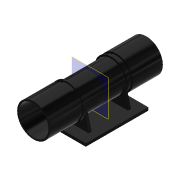
# Autodesk Inventor part: 00_Sensirion_Flowsensor
Saved by Autodesk Inventor 2019.4 (Build 234330000, 330)
## iProperties
Created: 2021-06-01
Part Number: 00_Sensirion_Flowsensor
Material: Generic
Document SubType Name: Modeling
Designer: diederichbenedict
Density: 1 g/cm^3
Appearance: Smooth - Black
Author: diederichbenedict
Autodesk Inventor part; units mm, degrees
ref_plane "YZ Plane" through (0, 0, 0) normal (1, 0, 0) x (0, 1, 0)
ref_plane "XZ Plane" through (0, 0, 0) normal (0, 1, 0) x (-1, 0, 0)
ref_plane "XY Plane" through (0, 0, 0) normal (0, 0, 1) x (1, 0, 0)
sketch "Sketch1" plane through (0, 0, 0) normal (0, 1, 0) x (-1, 0, 0)
  line L0 (0, 0) -> (0, 17.6)
  line L1 (0, 17.6) -> (0, 37.6)
  line L2 (0, 37.6) -> (11, 37.6)
  line L3 (11, 37.6) -> (11, 17.6)
  line L4 (11, 17.6) -> (9.9, 17.6)
  line L5 (9.9, 17.6) -> (9.9, 15.1)
  line L6 (9.9, 15.1) -> (11, 15.1)
  line L7 (11, 15.1) -> (11, 14.1)
  line L8 (11, 14.1) -> (9.9, 14.1)
  line L9 (9.9, 14.1) -> (9.9, 0)
  line L10 (9.9, 0) -> (0, 0)
  dimension "d0" = 17.6
  dimension "d1" = 20
  dimension "d2" = 11
  dimension "d3" = 20
  dimension "d4" = 9.9
  dimension "d6" = 2.5
  dimension "d7" = 1
  dimension "d8" = 0
  constraints: 22 end point, 6 perpendicular, 2 point on line, 1 parallel, 1 vertical
  measures "d0" distance of L0.start L0.end
  measures "d1" distance of L0.end L1.end
  measures "d2" distance of L1.end L2.end
  measures "d3" distance of L2.end L3.end
  measures "d4" distance of L9.end L0.start
  measures "d6" distance between parallel lines of L6 L4
  measures "d7" distance between parallel lines of L8 L6
  measures "d8" distance between parallel lines of L7 L3
revolve "Revolution1" add sketch "Sketch1" angle 360 about axis through (0, 0, 17.6) along (0, 0, 1)
sketch "Sketch2" plane through (0, 0, 37.6) normal (0, 0, 1) x (1, 0, 0)
  circle A0 centre (0, 0) radius 11 projected
  circle A1 centre (0, 0) radius 9.9
  constraints: 1 centre point, 1 coincident
extrude "Extrusion1" cut sketch "Sketch2" against normal through all draft -5 contours A1
mirror "Mirror1" about plane through (0, 0, 0) normal (0, 0, -1) of "Revolution1", "Extrusion1"
ref_plane "Work Plane1" through (0, 0, 0) normal (0, 0, -1) x (-1, 0, 0)
sketch "Sketch3" plane through (0, 0, 14.1) normal (0, 0, -1) x (-1, 0, 0)
  circle A0 centre (0, 0) radius 6.6104 projected
  circle A1 centre (0, 0) radius 9.9 projected
  circle A2 centre (0, 0) radius 9.9 projected
  line L0 (-9.9, 0) -> (-13.2646, -12.557)
  line L1 (-9.9, 0) -> (3.1, 0) construction
  line L2 (9.9, 0) -> (13.2646, -12.557)
  line L3 (9.9, 0) -> (22.9, 0) construction
  line L4 (13.2646, -12.557) -> (-13.2646, -12.557)
  dimension "d12" = 13
  dimension "d13" = 105
  dimension "d14" = 75
  constraints: 10 end point, 3 horizontal, 2 equal length, 2 point on circle
  measures "d12" distance of L0.start L0.end
  measures "d13" angle of L0 L1
  measures "d14" angle of L2 L3
extrude "Extrusion2" add sketch "Sketch3" along normal blind 2 contours L2 L4 L0 A1
mirror "Mirror2" about plane through (0, 0, 0) normal (0, 0, -1) of "Extrusion2"
sketch "Sketch4" plane through (-13.2646, -12.557, -14.1) normal (0, -1, 0) x (1, 0, 0)
  line L0 (26.5293, 0) -> (0, 0) projected
  line L1 (26.5293, 0) -> (26.5293, 2) projected
  line L2 (26.5293, 2) -> (0, 2) projected
  line L3 (0, 0) -> (0, 2) projected
  line L4 (26.5293, 28.2) -> (0, 28.2) projected
  line L5 (0, 28.2) -> (0, 26.2) projected
  line L6 (26.5293, 26.2) -> (0, 26.2) projected
  line L7 (26.5293, 28.2) -> (26.5293, 26.2) projected
  line L8 (31.3099, -6.7496) -> (-4.7806, -6.7496)
  line L9 (-4.7806, -6.7496) -> (-4.7806, 34.9496)
  line L10 (-4.7806, 34.9496) -> (31.3099, 34.9496)
  line L11 (31.3099, 34.9496) -> (31.3099, -6.7496)
  line L12 (31.3099, -6.7496) -> (-4.7806, 34.9496) construction
  line L13 (-4.7806, -6.7496) -> (31.3099, 34.9496) construction
  point P0 (13.2646, 14.1)
  constraints: 12 end point, 2 midpoint, 2 parallel, 1 horizontal, 1 perpendicular
extrude "Extrusion3" add sketch "Sketch4" along normal blind 2
body "Solid1"
